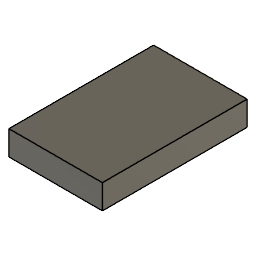
3dpcb (Autodesk Fusion 360 archive; units mm, degrees)
design "baterie"
part number: 2026-04-21-18-17-35-337
Autodesk Fusion 360 part; units mm, degrees
sketch "Sketch1" plane through (0, 0, 0) normal (0, 0, 1) x (1, 0, 0)
  line L0 (-9.7186, 14.8987) -> (11.2814, 14.8987)
  line L1 (11.2814, 14.8987) -> (11.2814, -17.6013)
  line L2 (-9.7186, 14.8987) -> (-9.7186, -17.6013)
  line L3 (-9.7186, -17.6013) -> (11.2814, -17.6013)
  dimension "d1" = 21
  dimension "d2" = 32.5
  dimension "d3" = 32.5
  constraint horizontal L0
  constraint perpendicular L0 L1
  constraint perpendicular L0 L2
  measures "d1" distance of L0.start L0.end
  measures "d2" distance of L0.end L1.end
  measures "d3" distance of L0.start L2.end
extrude "Extrude1" add sketch "Sketch1" along normal blind 5.5

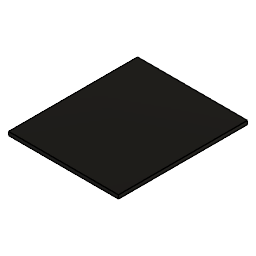
design "ecran"
part number: 2026-04-21-18-40-12-058
Autodesk Fusion 360 part; units mm, degrees
sketch "Sketch1" plane through (0, 0, 0) normal (0, 0, 1) x (1, 0, 0)
  line L0 (-15.606, 20.3886) -> (16.194, 20.3886)
  line L1 (16.194, 20.3886) -> (16.194, -16.9314)
  line L2 (16.194, -16.9314) -> (-15.606, -16.9314)
  line L3 (-15.606, -16.9314) -> (-15.606, 20.3886)
  dimension "d1" = 31.8
  dimension "d2" = 37.32
  constraint horizontal L0
  constraint perpendicular L0 L1
  constraint perpendicular L1 L2
  constraint perpendicular L0 L3
  measures "d1" distance of L0.start L0.end
  measures "d2" distance of L0.end L1.end
extrude "Extrude1" add sketch "Sketch1" along normal blind 1.05
